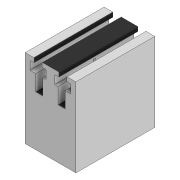
# Autodesk Inventor part: grippershapev2
Saved by Autodesk Inventor 2020.3 (Build 243373000, 373)
## iProperties
Created: 2020-05-25
Part Number: grippershapev2
Material: Generic
Document SubType Name: Modeling
Designer: Svend
Density: 1 g/cm^3
Appearance: Default
Author: Svend
Autodesk Inventor part; units mm, degrees
ref_plane "Work Plane2" through (-6.6, -11, -70) normal (0, 0, -1) x (0, 1, 0)
ref_plane "Work Plane3" through (21.95, -1.9, -8.0264) normal (0, 0, 1) x (1, 0, 0)
ref_plane "Work Plane4" through (21.95, -1.9, -8.0264) normal (0, 0, 1) x (1, 0, 0)
sketch "Sketch3" plane through (21.95, -1.9, -8.0264) normal (0, 0, 1) x (1, 0, 0)
  line L0 (-6.75, 7.95) -> (-6.75, 1.35) projected
  line L1 (-6.75, 1.35) -> (-6.55, 1.15) projected
  line L2 (-6.55, 1.15) -> (-1.7, 1.15) projected
  line L3 (-1.7, 1.15) -> (-1.7, -12.85) projected
  line L4 (-4.0364, -12.85) -> (-4.0294, -12.85) projected
  line L5 (-2.65, -12.85) -> (-4.0294, -12.85) projected
  line L6 (-1.7, -12.85) -> (-2.65, -12.85) projected
  line L7 (-2.65, -12.85) -> (-2.65, -0.85) projected
  line L8 (-6.75, 7.95) -> (-6.55, 8.15) projected
  line L9 (-3.2, 8.15) -> (-6.55, 8.15) projected
  line L10 (-3.2, 12.75) -> (-3.2, 8.15) projected
  line L11 (-3.2, 12.75) -> (-3, 12.95) projected
  line L12 (3.1, 12.95) -> (-3, 12.95) projected
  line L13 (3.1, 12.95) -> (3.3, 12.75) projected
  line L14 (3.3, 8.15) -> (3.3, 12.75) projected
  line L15 (6.65, 8.15) -> (3.3, 8.15) projected
  line L16 (6.65, 8.15) -> (6.85, 7.95) projected
  line L17 (6.85, 1.35) -> (6.85, 7.95) projected
  line L18 (6.85, 1.35) -> (6.65, 1.15) projected
  line L19 (1.8, 1.15) -> (6.65, 1.15) projected
  line L20 (1.8, -12.65) -> (1.8, 1.15) projected
  line L21 (1.8, -12.85) -> (1.8, -12.65) projected
  line L22 (-1.7, -12.85) -> (1.8, -12.85) projected
  line L23 (-4.0294, -12.85) -> (-4.125, 1.15)
  line L24 (-7.05, 1.2257) -> (-7.05, 8.0743)
  line L25 (-7.05, 8.0743) -> (-6.6743, 8.45)
  line L26 (-6.6743, 8.45) -> (-3.5, 8.45)
  line L27 (-3.5, 8.45) -> (-3.5, 12.8743)
  line L28 (-3.5, 12.8743) -> (-3.1243, 13.25)
  line L29 (-3.1243, 13.25) -> (3.2243, 13.25)
  line L30 (3.2243, 13.25) -> (3.6, 12.8743)
  line L31 (3.6, 12.8743) -> (3.6, 8.45)
  line L32 (3.6, 8.45) -> (6.7743, 8.45)
  line L33 (6.7743, 8.45) -> (7.15, 8.0743)
  line L34 (7.15, 8.0743) -> (7.15, 1.2257)
  line L35 (7.15, 1.2257) -> (6.7743, 0.85)
  line L36 (6.7743, 0.85) -> (2.1, 0.85)
  line L37 (2.1, 0.85) -> (2.1, -12.65)
  line L38 (2.1, -12.65) -> (2.1, -13.15)
  line L39 (2.1, -13.15) -> (-2, -13.15)
  line L40 (-2, -13.15) -> (-2, 0.85)
  line L41 (-2, 0.85) -> (-6.6743, 0.85)
  line L42 (-6.6743, 0.85) -> (-7.05, 1.2257)
  line L43 (-4.1273, -13.15) -> (-4.2253, 1.1991)
  line L44 (-2, -13.15) -> (-4.1273, -13.15)
  line L45 (-13.925, -1.05) -> (-8.025, -1.05) projected
  line L46 (-10.975, -1.05) -> (-10.975, -12.3939)
  line L47 (-15.2, 7.95) -> (-15.2, 1.35)
  line L48 (-15.2, 1.35) -> (-15.4, 1.15)
  line L49 (-15.4, 1.15) -> (-20.25, 1.15)
  line L50 (-20.25, 1.15) -> (-20.25, -12.85)
  line L51 (-17.9136, -12.85) -> (-17.9206, -12.85)
  line L52 (-19.3, -12.85) -> (-17.9206, -12.85)
  line L53 (-20.25, -12.85) -> (-19.3, -12.85)
  line L54 (-19.3, -12.85) -> (-19.3, -0.85)
  line L55 (-15.2, 7.95) -> (-15.4, 8.15)
  line L56 (-18.75, 8.15) -> (-15.4, 8.15)
  line L57 (-18.75, 12.75) -> (-18.75, 8.15)
  line L58 (-18.75, 12.75) -> (-18.95, 12.95)
  line L59 (-25.05, 12.95) -> (-18.95, 12.95)
  line L60 (-25.05, 12.95) -> (-25.25, 12.75)
  line L61 (-25.25, 8.15) -> (-25.25, 12.75)
  line L62 (-28.6, 8.15) -> (-25.25, 8.15)
  line L63 (-28.6, 8.15) -> (-28.8, 7.95)
  line L64 (-28.8, 1.35) -> (-28.8, 7.95)
  line L65 (-28.8, 1.35) -> (-28.6, 1.15)
  line L66 (-23.75, 1.15) -> (-28.6, 1.15)
  line L67 (-23.75, -12.65) -> (-23.75, 1.15)
  line L68 (-23.75, -12.85) -> (-23.75, -12.65)
  line L69 (-20.25, -12.85) -> (-23.75, -12.85)
  line L70 (-17.9206, -12.85) -> (-17.825, 1.15)
  line L71 (-14.9, 1.2257) -> (-14.9, 8.0743)
  line L72 (-14.9, 8.0743) -> (-15.2757, 8.45)
  line L73 (-15.2757, 8.45) -> (-18.45, 8.45)
  line L74 (-18.45, 8.45) -> (-18.45, 12.8743)
  line L75 (-18.45, 12.8743) -> (-18.8257, 13.25)
  line L76 (-18.8257, 13.25) -> (-25.1743, 13.25)
  line L77 (-25.1743, 13.25) -> (-25.55, 12.8743)
  line L78 (-25.55, 12.8743) -> (-25.55, 8.45)
  line L79 (-25.55, 8.45) -> (-28.7243, 8.45)
  line L80 (-28.7243, 8.45) -> (-29.1, 8.0743)
  line L81 (-29.1, 8.0743) -> (-29.1, 1.2257)
  line L82 (-29.1, 1.2257) -> (-28.7243, 0.85)
  line L83 (-28.7243, 0.85) -> (-24.05, 0.85)
  line L84 (-24.05, 0.85) -> (-24.05, -12.65)
  line L85 (-24.05, -12.65) -> (-24.05, -13.15)
  line L86 (-24.05, -13.15) -> (-19.95, -13.15)
  line L87 (-19.95, -13.15) -> (-19.95, 0.85)
  line L88 (-19.95, 0.85) -> (-15.2757, 0.85)
  line L89 (-15.2757, 0.85) -> (-14.9, 1.2257)
  line L90 (-17.8227, -13.15) -> (-17.7247, 1.1991)
  line L91 (-19.95, -13.15) -> (-17.8227, -13.15)
  line L92 (-33.425, 12.25) -> (11.575, 12.25)
  line L93 (11.575, 12.25) -> (11.575, -57.75)
  line L94 (11.575, -57.75) -> (-33.425, -57.75)
  line L95 (-33.425, -57.75) -> (-33.425, 12.25)
  point P0 (-21.95, 1.9)
  point P1 (-10.925, -52.6184)
  point P2 (-10.925, -57.75)
  point P3 (-3.5, 12.25)
  point P4 (-18.45, 12.25)
  point P5 (-17.727, 0.85)
  point P6 (-25.55, 12.25)
  point P7 (3.6, 12.25)
  point P8 (-4.223, 0.85)
  dimension "d18" = 0.3
  dimension "d19" = 0.1
  dimension "d20" = 1
  dimension "d21" = 45
  dimension "d22" = 70
  constraints: 144 end point, 45 symmetric about line, 3 midpoint, 3 parallel, 2 horizontal, 1 perpendicular, 1 vertical, 1 vertical alignment, 18 other
  measures "d18" distance between parallel lines of L0 L24
  measures "d19" distance between parallel lines of L23 L43
  measures "d20" distance between parallel lines of L76 L92
  measures "d21" distance of L93.end L94.end
  measures "d22" distance between parallel lines of L92 L94
extrude "Extrusion2" add sketch "Sketch3" against normal blind 70 contours L43 L44 L39 L38 L37 L36 L35 L34 L33 L32 L31 L92 L93 L94 L95 L78 L79 L80 L81 L82 L83 L84 L85 L86 L91 L90 L88 L89 L71 L72 L73 L74 L27 L26 L25 L24 L42 L41
sketch "Sketch4" plane through (-11.475, -59.65, -8.0264) normal (0, -1, 0) x (1, 0, 0)
  line L0 (0, 0) -> (45, 0) projected
  line L1 (0, 0) -> (0, -70) projected
  line L2 (45, -70) -> (0, -70) projected
  line L3 (45, 0) -> (45, -70) projected
  circle A0 centre (22.5, -35) radius 9
  point P0 (11.475, 8.0264)
  point P1 (22.5, 0)
  point P2 (45, -35)
  dimension "d25" = 18
  constraints: 2 midpoint, 1 centre point, 1 horizontal alignment, 1 vertical alignment
  measures "d25" diameter of A0
ref_plane "Work Plane5" through (1.75, -2.8, -26.5932) normal (0, 1, 0) x (0, 0, 1)
extrude "Extrusion3" cut sketch "Sketch4" against normal blind 57.25 contours A0
sketch "Sketch5" plane through (-11.475, -59.65, -8.0264) normal (0, -1, 0) x (1, 0, 0)
  circle A0 centre (22.5, -35) radius 9 projected
  circle A1 centre (22.5, -35) radius 4
  point P0 (11.475, 8.0264)
  dimension "d28" = 8
  constraints: 1 centre point, 1 coincident
  measures "d28" diameter of A1
extrude "Extrusion4" cut sketch "Sketch5" against normal blind 61 contours A1
ref_plane "Work Plane6" through (1.2787, -51.0682, -52.9264) normal (0, 0, -1) x (0, 1, 0)
ref_plane "Work Plane7" through (10.975, -59.9, -43.0264) normal (0, -1, 0) x (1, 0, 0)
sketch "Sketch10" plane through (10.975, -59.9, -43.0264) normal (0, -1, 0) x (1, 0, 0)
  line L0 (29.6, 9.9) -> (-9, 9.9) projected
  arc A0 (-9, 9.9) -> (-10, 8.9) centre (-9, 8.9) ccw projected
  line L1 (-10, 8.9) -> (-10, -8.9) projected
  arc A1 (30.6, 8.9) -> (29.6, 9.9) centre (29.6, 8.9) ccw projected
  line L2 (30.6, -8.9) -> (30.6, 8.9) projected
  arc A2 (29.6, -9.9) -> (30.6, -8.9) centre (29.6, -8.9) ccw projected
  line L3 (-9, -9.9) -> (29.6, -9.9) projected
  arc A3 (-10, -8.9) -> (-9, -9.9) centre (-9, -8.9) ccw projected
  line L4 (-10, 8.9) -> (-10, -8.9) projected
  line L5 (-10.2, -12) -> (-10.2, 30.5)
  line L6 (-10.2, 30.5) -> (10.2, 30.5)
  line L7 (10.2, 30.5) -> (10.2, -12)
  line L8 (10.2, -12) -> (-10.2, -12)
  circle A4 centre (0, 0) radius 9 projected
  circle A5 centre (0.05, 0) radius 9 projected
  line L9 (-22.45, 35) -> (-22.45, -35) projected
  line L10 (22.55, 35) -> (22.55, -35) projected
  line L11 (-22.45, 35) -> (22.55, 35) projected
  line L12 (22.55, -35) -> (-22.45, -35) projected
  point P0 (-10.975, 43.0264)
  point P1 (0, -12)
  dimension "d45" = 20.4
  dimension "d46" = 12
  dimension "d47" = 30.5
  constraints: 8 end point, 2 parallel, 1 midpoint, 1 perpendicular
  measures "d45" distance between parallel lines of L7 L5
  measures "d46" distance from line of L8 A4.centre
  measures "d47" distance from line of L6 A4.centre
extrude "Extrusion12" cut sketch "Sketch10" against normal blind 43 contours L7 L3 A3 L1 A0 L0 | L0 A0 L1 A3 L3 L7 L8 L5 L6 | A4 A5 | A4 A5 | A5 A4
fillet "Fillet10" radius 0.2 4 edges at (25.55, 10.35, -43.0264) (18.45, 10.35, -43.0264) (3.5, 10.35, -43.0264) (-3.6, 10.35, -43.0264)
chamfer "Chamfer5" distance 0.5 angle 45 4 edges at (19.4565, -15.05, -46.1745) (19.4565, -15.05, -39.8784) (2.025, -15.05, -43.0264) (7.025, -2.4, -43.0264)
body "Solid2"
